Autodesk Fusion 360 part; units mm, degrees
(part 2 of 2)
sketch "bottom_shell" plane through (0, 0, -4.4) normal (0, 0, 1) x (1, 0, 0) in component "diag_up_bottom_noVM"
  circle A0 centre (49, 51) radius 1.5875 construction
  line L0 (1, 0) -> (52, 0) construction
  line L1 (0, 1) -> (0, 54) construction
  line L2 (53, 1) -> (53, 54) construction
  circle A1 centre (4, 51) radius 1.5875 construction
  line L3 (52, 55) -> (1, 55) construction
  line L4 (-7.5, 57.5) -> (60.5, 57.5)
  line L5 (63.5, 54.5) -> (63.5, 3)
  line L6 (60.5, 0) -> (-7.5, 0)
  line L7 (-10.5, 3) -> (-10.5, 54.5)
  arc A2 (-7.5, 57.5) -> (-10.5, 54.5) centre (-7.5, 54.5) ccw
  arc A3 (63.5, 54.5) -> (60.5, 57.5) centre (60.5, 54.5) ccw
  arc A4 (60.5, 0) -> (63.5, 3) centre (60.5, 3) ccw
  arc A5 (-10.5, 3) -> (-7.5, 0) centre (-7.5, 3) ccw
  arc A6 (61.5, 54.5) -> (60.5, 55.5) centre (60.5, 54.5) ccw
  line L8 (-7.5, 55.5) -> (60.5, 55.5)
  arc A7 (-7.5, 55.5) -> (-8.5, 54.5) centre (-7.5, 54.5) ccw
  line L9 (-8.5, 3) -> (-8.5, 54.5)
  arc A8 (-8.5, 3) -> (-7.5, 2) centre (-7.5, 3) ccw
  line L10 (60.5, 2) -> (-7.5, 2)
  arc A9 (60.5, 2) -> (61.5, 3) centre (60.5, 3) ccw
  line L11 (61.5, 54.5) -> (61.5, 3)
  arc A10 (62.3, 54.5) -> (60.5, 56.3) centre (60.5, 54.5) ccw
  line L12 (-7.5, 56.3) -> (60.5, 56.3)
  arc A11 (-7.5, 56.3) -> (-9.3, 54.5) centre (-7.5, 54.5) ccw
  line L13 (-9.3, 3) -> (-9.3, 54.5)
  arc A12 (-9.3, 3) -> (-7.5, 1.2) centre (-7.5, 3) ccw
  arc A13 (60.5, 1.2) -> (62.3, 3) centre (60.5, 3) ccw
  line L14 (62.3, 54.5) -> (62.3, 3)
  circle A14 centre (49, 51) radius 1.75
  circle A15 centre (49, 51) radius 3.5
  circle A16 centre (49, 51) radius 4.25
  circle A17 centre (4, 51) radius 1.75
  circle A18 centre (4, 51) radius 3.5
  circle A19 centre (4, 51) radius 4.25
  circle A20 centre (-4.25, 6.25) radius 1.75
  circle A21 centre (-4.25, 6.25) radius 3
  circle A22 centre (-4.25, 6.25) radius 4
  line L15 (-0.3, 2) -> (-0.3, 0)
  line L16 (53.3, 2) -> (53.3, 0)
  circle A23 centre (57.25, 6.25) radius 1.75
  circle A24 centre (57.25, 6.25) radius 3
  circle A25 centre (57.25, 6.25) radius 4
  line L17 (60.5, 1.2) -> (53, 1.2)
  line L18 (0, 1.2) -> (-7.5, 1.2)
  line L19 (26.5, 55) -> (26.5, 2) construction
  line L20 (-5.7027, 21) -> (58.2376, 21) construction
  line L21 (-2, 22.5) -> (2, 22.5)
  line L22 (2, 22.5) -> (2, 19.5)
  line L23 (2, 19.5) -> (-2, 19.5)
  line L24 (-2, 19.5) -> (-2, 22.5)
  line L25 (-0.3, 22.5) -> (-0.3, 19.5)
  line L26 (51, 22.5) -> (55, 22.5)
  line L27 (55, 22.5) -> (55, 19.5)
  line L28 (55, 19.5) -> (51, 19.5)
  line L29 (51, 19.5) -> (51, 22.5)
  line L30 (54, 22.5) -> (53.3, 22.5)
  line L31 (53.3, 22.5) -> (53.3, 19.5)
  line L32 (53.3, 19.5) -> (54, 19.5)
  line L33 (-8.5, 22.5) -> (-8.5, 22.5)
  line L34 (-2, 22.5) -> (-2, 22.5)
  line L35 (-2, 19.5) -> (-8.5, 19.5)
  line L36 (-8.5, 19.5) -> (-8.5, 19.5)
  line L37 (-2, 19.5) -> (-2, 19.5)
  line L38 (55, 22.5) -> (61.5, 22.5)
  line L39 (55, 19.5) -> (61.5, 19.5)
  line L40 (-2, 22.5) -> (-8.5, 22.5)
  line L41 (-4.25, 6.25) -> (-4.25, 10.25) construction
  line L42 (-4.25, 6.25) -> (-0.25, 6.25) construction
  line L43 (57.25, 6.25) -> (53.25, 6.25) construction
  line L44 (57.25, 6.25) -> (57.25, 10.25) construction
  line L45 (57.25, 10.25) -> (61.5, 10.25)
  line L46 (53.3, 2) -> (53.3, 5.6195)
  line L47 (-4.25, 10.25) -> (-8.5, 10.25)
  line L48 (4, 51) -> (8.25, 51) construction
  line L49 (4, 51) -> (-0.25, 51) construction
  line L50 (49, 51) -> (53.25, 51) construction
  line L51 (49, 51) -> (44.75, 51) construction
  line L52 (44.75, 51) -> (44.75, 55.5)
  line L53 (53.25, 51) -> (53.25, 55.5)
  line L54 (8.25, 51) -> (8.25, 55.5)
  line L55 (-0.25, 51) -> (-0.25, 55.5)
  line L56 (-0.3, 2) -> (-0.3, 5.6195)
  point P0 (49, 51)
  point P1 (49, 51)
  dimension "d47" = 57.5
  dimension "d48" = 3
  dimension "d49" = 10.5
  dimension "d50" = 74
  dimension "d51" = 2
  dimension "d53" = 3.5
  dimension "d54" = 7
  dimension "d56" = 3.5
  dimension "d57" = 7
  dimension "d58" = 8.5
  dimension "d59" = 4.25
  dimension "d60" = 4.25
  dimension "d61" = 3.5
  dimension "d62" = 6
  dimension "d63" = 8
  dimension "d64" = 0.3
  dimension "d65" = 0.3
  dimension "d66" = 3.5
  dimension "d67" = 4.25
  dimension "d68" = 4.25
  dimension "d69" = 6
  dimension "d70" = 8
  dimension "d71" = 8.5
  dimension "d72" = 1.2
  dimension "d85" = 19
  dimension "d86" = 4
  dimension "d87" = 3
  dimension "d88" = 0.3
  dimension "d89" = 4
  dimension "d90" = 3
  dimension "d91" = 0.3
  constraint horizontal L4
  constraint vertical L5
  constraint horizontal L6
  constraint vertical L7
  constraint collinear L0 L6
  constraint tangent L4 A2
  constraint tangent L7 A2
  constraint tangent L4 A3
  constraint tangent L5 A3
  constraint equal A2 A3
  constraint tangent L5 A4
  constraint tangent L6 A4
  constraint equal A2 A4
  constraint tangent L6 A5
  constraint tangent L7 A5
  constraint equal A2 A5
  constraint coincident P0 A0.centre
  constraint concentric A14 A15
  constraint concentric A15 A16
  constraint concentric A1 A17
  constraint concentric A1 A18
  constraint concentric A17 A19
  constraint concentric A20 A21
  constraint concentric A20 A22
  constraint coincident L10 L15.start
  constraint coincident L6 L15.end
  constraint perpendicular L6 L15
  constraint coincident L10 L16.start
  constraint coincident L6 L16.end
  constraint perpendicular L6 L16
  constraint concentric A23 A24
  constraint concentric A24 A25
  constraint concentric A3 A10
  constraint parallel L4 L12
  constraint concentric A2 A11
  constraint parallel L7 L13
  constraint concentric A5 A12
  constraint parallel L6 L17
  constraint concentric A4 A13
  constraint parallel L5 L14
  constraint tangent A10 L14
  constraint tangent A13 L17
  constraint tangent A10 L12
  constraint tangent A13 L14
  constraint tangent L12 A11
  constraint tangent A11 L13
  constraint tangent A12 L17
  constraint tangent L13 A12
  constraint coincident L2 L17.end
  constraint coincident L1 L18.start
  constraint collinear L17 L18
  constraint midpoint L3 L19.start
  constraint midpoint L10 L19.end
  constraint perpendicular L2 L20
  constraint horizontal L21
  constraint vertical L22
  constraint horizontal L23
  constraint vertical L24
  constraint symmetric L20 L21 L23
  constraint symmetric L1 L22 L24
  constraint coincident L21 L25.start
  constraint coincident L23 L25.end
  constraint perpendicular L23 L25
  constraint horizontal L26
  constraint vertical L27
  constraint horizontal L28
  constraint vertical L29
  constraint horizontal L30
  constraint vertical L31
  constraint horizontal L32
  constraint coincident L28 L31.end
  constraint coincident L26 L30.start
  constraint symmetric L20 L26 L28
  constraint symmetric L2 L27 L29
  constraint coincident L9 L33.start
  constraint horizontal L35
  constraint coincident L9 L35.end
  constraint coincident L11 L38.end
  constraint perpendicular L11 L38
  constraint coincident L11 L39.end
  constraint perpendicular L11 L39
  constraint perpendicular L9 L40
  constraint coincident A20.centre A21.centre
  constraint coincident A22 L41.end
  constraint vertical L41
  constraint coincident A22 L42.end
  constraint perpendicular L41 L42
  constraint coincident A23.centre A24.centre
  constraint coincident A25 L43.end
  constraint perpendicular L19 L43
  constraint coincident A25 L44.end
  constraint perpendicular L43 L44
  constraint coincident L11 L45.end
  constraint tangent A25 L45
  constraint coincident A25 L46.end
  constraint perpendicular L10 L46
  constraint coincident L9 L47.end
  constraint tangent A22 L47
  constraint coincident A1.centre A17.centre
  constraint coincident A19 L48.end
  constraint horizontal L48
  constraint coincident A19 L49.end
  constraint perpendicular L1 L49
  constraint coincident P1 P0
  constraint coincident A16 L50.end
  constraint coincident A16 L51.end
  constraint horizontal L51
  constraint coincident L8 L52.end
  constraint tangent A16 L52
  constraint coincident L8 L53.end
  constraint tangent A16 L53
  constraint perpendicular L8 L53
  constraint coincident L8 L54.end
  constraint tangent A19 L54
  constraint coincident L8 L55.end
  constraint tangent A19 L55
  constraint coincident A22 L56.end
  constraint perpendicular L10 L56
  measures "d47" distance of L4 L6
  measures "d48" radius of A2
  measures "d49" distance of L1 L7
  measures "d50" distance of L5 L7
  measures "d53" diameter of A14
  measures "d54" diameter of A15
  measures "d56" diameter of A17
  measures "d57" diameter of A18
  measures "d58" diameter of A19
  measures "d59" distance of L1 A20.centre
  measures "d60" distance of L10 A20.centre
  measures "d61" diameter of A20
  measures "d62" diameter of A21
  measures "d63" diameter of A22
  measures "d64" distance of L1 L15
  measures "d65" distance of L2 L16
  measures "d66" diameter of A23
  measures "d67" distance of L2 A23.centre
  measures "d68" distance of L10 A23.centre
  measures "d69" diameter of A24
  measures "d70" diameter of A25
  measures "d71" diameter of A16
  measures "d72" distance of L7 L13
  measures "d85" distance of L10 L20
  measures "d86" distance of L22 L24
  measures "d87" distance of L21 L23
  measures "d88" distance of L1 L25
  measures "d89" distance of L27 L29
  measures "d90" distance of L26 L28
  measures "d91" distance of L2 L31
extrude "Extrude1'" add sketch "bottom_shell" against normal blind 2 separate body contours L4 L5 L6 L7 A2 A3 A4 A5 A10 L12 A11 L13 A12 A13 L14 L15 L16 L17 L18 | L6 L10 L15 L16 | A6 L8 A7 L9 A8 L10 A9 L11 A10 L12 A11 L13 A12 A13 L14 L15 L16 L17 L18 | A6 L8 A7 L9 L10 L11 A16 A19 A22 A25 L21 L22 L23 L26 L28 L29 L30 L32 L35 L38 L39 L40 L45 L46 L47 L52 L53 L54 L55 L56 | L9 A8 L10 A22 L47 L56 | L10 A9 L11 A25 L45 L46 | A22 | A25 | L9 L24 L35 L40 | L11 L27 L38 L39 | L21 L23 L24 L25 | L26 L27 L28 L30 L31 L32 | L21 L22 L23 L25 | L26 L28 L29 L31 | L8 A19 L54 L55 | L8 A16 L52 L53 | A19 | A16 makes body 2 in component "diag_up_bottom_noVM"
extrude "Extrude2'" add sketch "bottom_shell" along normal blind 1 contours L6 L10 L15 L16 bodies 2 in component "diag_up_bottom_noVM"
extrude "Extrude3'" add sketch "bottom_shell" along normal blind 9.7 contours A6 L8 A7 L9 A8 L10 A9 L11 A10 L12 A11 L13 A12 A13 L14 L15 L16 L17 L18 bodies 2 in component "diag_up_bottom_noVM"
extrude "Extrude4'" add sketch "bottom_shell" along normal blind 8.7 contours L4 L5 L6 L7 A2 A3 A4 A5 A10 L12 A11 L13 A12 A13 L14 L15 L16 L17 L18 bodies 2 in component "diag_up_bottom_noVM"
extrude "Extrude5'" add sketch "bottom_shell" along normal blind 2.8 contours L21 L22 L23 L25 | L26 L28 L29 L31 | L8 A19 L54 L55 | L8 A16 L52 L53 | A19 | A16 | A15 | A18 bodies 2 in component "diag_up_bottom_noVM"
extrude "Extrude6'" add sketch "bottom_shell" along normal blind 4.4 contours L9 A8 L10 A22 L47 L56 | L10 A9 L11 A25 L45 L46 | A22 | A25 | L9 L24 L35 L40 | L11 L27 L38 L39 | L21 L23 L24 L25 | L26 L27 L28 L30 L31 L32 | A21 | A24 bodies 2 in component "diag_up_bottom_noVM"
fillet "Fillet6" radius 1 10 edges at (8.25, 55.5, -3) (-0.25, 55.5, -3) (-8.5, 22.5, -2.2) (-8.5, 19.5, -2.2) (-8.5, 10.25, -2.2) (61.5, 10.25, -2.2) (61.5, 19.5, -2.2) (61.5, 22.5, -2.2) (53.25, 55.5, -3) (44.75, 55.5, -3) on bodies 2 in component "diag_up_bottom_noVM"
chamfer "Chamfer2" distance 1 angle 45 18 edges at (-5.875, 10.25, 0) (-8.2071, 10.5429, 0) (-1.2068, 8.846, 0) (-0.3, 3.8098, 0) (4, 46.75, -1.6) (8.25, 52.75, -1.6) (8.5429, 55.2071, -1.6) (-0.5429, 55.2071, -1.6) (-0.25, 52.75, -1.6) (44.75, 52.75, -1.6) (49, 46.75, -1.6) (53.25, 52.75, -1.6) (53.5429, 55.2071, -1.6) (44.4571, 55.2071, -1.6) (58.875, 10.25, 0) (54.2068, 8.846, 0) (61.2071, 10.5429, 0) (53.3, 3.8098, 0) on bodies 2 in component "diag_up_bottom_noVM"
fillet "Fillet7" radius 0.5 8 edges at (-0.3, 22.5, -0.8) (2, 22.5, -3) (2, 19.5, -3) (-0.3, 19.5, -0.8) (53.3, 22.5, -0.8) (53.3, 19.5, -0.8) (51, 19.5, -3) (51, 22.5, -3) on bodies 2 in component "diag_up_bottom_noVM"
fillet "Fillet8" radius 0.5 42 edges at (54.2068, 8.846, -4.4) (58.875, 10.25, -4.4) (61.2071, 10.5429, -4.4) (61.5, 14.875, -4.4) (61.2071, 19.2071, -4.4) (56, 19.5, -4.4) (51.1464, 19.6464, -4.4) (51, 21, -4.4) (51.1464, 22.3536, -4.4) (56, 22.5, -4.4) (61.2071, 22.7929, -4.4) (61.5, 39, -4.4) (61.2071, 55.2071, -4.4) (57.375, 55.5, -4.4) (53.5429, 55.2071, -4.4) (53.25, 52.75, -4.4) (49, 46.75, -4.4) (44.75, 52.75, -4.4) (44.4571, 55.2071, -4.4) (26.5, 55.5, -4.4) (8.5429, 55.2071, -4.4) (8.25, 52.75, -4.4) (4, 46.75, -4.4) (-0.25, 52.75, -4.4) (-0.5429, 55.2071, -4.4) (-4.375, 55.5, -4.4) (-8.2071, 55.2071, -4.4) (-8.5, 39, -4.4) (-8.2071, 22.7929, -4.4) (-3, 22.5, -4.4) (1.8536, 22.3536, -4.4) (2, 21, -4.4) (1.8536, 19.6464, -4.4) (-3, 19.5, -4.4) (-8.2071, 19.2071, -4.4) (-8.5, 14.875, -4.4) (-8.2071, 10.5429, -4.4) (-5.875, 10.25, -4.4) (-1.2068, 8.846, -4.4) (-0.3, 3.8098, -4.4) (53.3, 3.8098, -4.4) (26.5, 2, -4.4) on bodies 2 in component "diag_up_bottom_noVM"
fillet "Fillet9" radius 0.5 3 edges at (-0.3, 0, 0.45) (26.5, 0, -3.4) (53.3, 0, 0.45) on bodies 2 in component "diag_up_bottom_noVM"
fillet "Fillet10" radius 0.5 2 edges at (-0.3, 2, 2.15) (53.3, 2, 2.15) on bodies 2 in component "diag_up_bottom_noVM"
fillet "Fillet11" radius 0.5 2 edges at (4, 55.5, -1.6) (49, 55.5, -1.6) on bodies 2 in component "diag_up_bottom_noVM"
fillet "Fillet12" radius 0.5 2 edges at (-8.5, 21, 0) (61.5, 21, 0) on bodies 2 in component "diag_up_bottom_noVM"
ref_plane "WorkPlane1" through (0, 0, 8) normal (0, 0, 1) x (1, 0, 0) in component "diag_up_top_noVM"
sketch "top shell" plane through (0, 0, 8) normal (0, 0, 1) x (1, 0, 0) in component "diag_up_top_noVM"
  line L0 (2.8575, 28.7338) -> (4.2862, 28.7338) construction
  line L1 (1.4287, 28.7338) -> (2.8575, 28.7338) construction
  line L2 (1.4287, 8.4138) -> (1.4287, 28.7338) construction
  line L3 (4.2862, 28.7338) -> (10.6363, 28.7338) construction
  line L4 (10.6363, 28.7338) -> (10.6363, 20.6376) construction
  line L5 (10.6363, 20.6376) -> (10.6363, 16.5099) construction
  line L6 (10.6363, 16.5099) -> (10.6363, 8.4138) construction
  line L7 (10.6363, 8.4138) -> (4.2862, 8.4138) construction
  line L8 (4.2862, 8.4138) -> (2.8575, 8.4138) construction
  line L9 (2.8575, 8.4138) -> (1.4287, 8.4138) construction
  line L10 (16.84, 48.2537) -> (16.84, 54.6038) construction
  line L11 (16.84, 54.6038) -> (24.9362, 54.6038) construction
  line L12 (16.84, 46.825) -> (16.84, 48.2537) construction
  line L13 (16.84, 45.3962) -> (16.84, 46.825) construction
  line L14 (37.16, 45.3962) -> (16.84, 45.3962) construction
  line L15 (37.16, 46.825) -> (37.16, 45.3962) construction
  line L16 (37.16, 48.2537) -> (37.16, 46.825) construction
  line L17 (37.16, 54.6038) -> (37.16, 48.2537) construction
  line L18 (29.0638, 54.6038) -> (37.16, 54.6038) construction
  line L19 (24.9362, 54.6038) -> (29.0638, 54.6038) construction
  line L20 (46.2537, 45.16) -> (52.6038, 45.16) construction
  line L21 (44.825, 45.16) -> (46.2537, 45.16) construction
  line L22 (43.3962, 45.16) -> (44.825, 45.16) construction
  line L23 (43.3962, 24.84) -> (43.3962, 45.16) construction
  line L24 (52.6038, 45.16) -> (52.6038, 37.0638) construction
  line L25 (52.6038, 37.0638) -> (52.6038, 32.9362) construction
  line L26 (52.6038, 32.9362) -> (52.6038, 24.84) construction
  line L27 (52.6038, 24.84) -> (46.2537, 24.84) construction
  line L28 (46.2537, 24.84) -> (44.825, 24.84) construction
  line L29 (44.825, 24.84) -> (43.3962, 24.84) construction
  line L30 (43.3962, 23.62) -> (44.825, 23.62) construction
  line L31 (44.825, 23.62) -> (46.2537, 23.62) construction
  line L32 (46.2537, 23.62) -> (52.6038, 23.62) construction
  line L33 (52.6038, 23.62) -> (52.6038, 17.27) construction
  line L34 (43.3962, 8.38) -> (43.3962, 23.62) construction
  line L35 (44.825, 8.38) -> (43.3962, 8.38) construction
  line L36 (46.2537, 8.38) -> (44.825, 8.38) construction
  line L37 (52.6038, 8.38) -> (46.2537, 8.38) construction
  line L38 (52.6038, 14.73) -> (52.6038, 8.38) construction
  line L39 (52.6038, 17.27) -> (52.6038, 14.73) construction
  circle A0 centre (49, 51) radius 1.5875 construction
  circle A1 centre (57.25, 6.25) radius 1.75 construction
  circle A2 centre (-4.25, 6.25) radius 1.75 construction
  circle A3 centre (4, 51) radius 1.5875 construction
  line L40 (0, 1) -> (0, 54) construction
  line L41 (53, 1) -> (53, 54) construction
  line L42 (60.5, 2) -> (-7.5, 2)
  line L43 (60.5, 0) -> (-7.5, 0)
  arc A4 (-10.5, 3) -> (-7.5, 0) centre (-7.5, 3) ccw
  arc A5 (-8.5, 3) -> (-7.5, 2) centre (-7.5, 3) ccw
  line L44 (-8.5, 3) -> (-8.5, 54.5)
  line L45 (-10.5, 3) -> (-10.5, 54.5)
  arc A6 (-7.5, 55.5) -> (-8.5, 54.5) centre (-7.5, 54.5) ccw
  arc A7 (-7.5, 57.5) -> (-10.5, 54.5) centre (-7.5, 54.5) ccw
  line L46 (-7.5, 57.5) -> (60.5, 57.5)
  line L47 (-7.5, 55.5) -> (60.5, 55.5)
  arc A8 (63.5, 54.5) -> (60.5, 57.5) centre (60.5, 54.5) ccw
  arc A9 (61.5, 54.5) -> (60.5, 55.5) centre (60.5, 54.5) ccw
  line L48 (63.5, 54.5) -> (63.5, 3)
  line L49 (61.5, 54.5) -> (61.5, 3)
  arc A10 (60.5, 0) -> (63.5, 3) centre (60.5, 3) ccw
  arc A11 (60.5, 2) -> (61.5, 3) centre (60.5, 3) ccw
  line L50 (0, 2) -> (0, 0)
  line L51 (53, 2) -> (53, 0)
  arc A12 (62.7, 54.5) -> (60.5, 56.7) centre (60.5, 54.5) ccw
  line L52 (-7.5, 56.7) -> (60.5, 56.7)
  arc A13 (-7.5, 56.7) -> (-9.7, 54.5) centre (-7.5, 54.5) ccw
  line L53 (-9.7, 3) -> (-9.7, 54.5)
  arc A14 (-9.7, 3) -> (-7.5, 0.8) centre (-7.5, 3) ccw
  arc A15 (60.5, 0.8) -> (62.7, 3) centre (60.5, 3) ccw
  line L54 (62.7, 54.5) -> (62.7, 3)
  line L55 (60.5, 0.8) -> (53, 0.8)
  line L56 (0, 0.8) -> (-7.5, 0.8)
  circle A16 centre (4, 51) radius 1.25
  circle A17 centre (57.25, 6.25) radius 1.25
  circle A18 centre (-4.25, 6.25) radius 1.25
  circle A19 centre (49, 51) radius 1.25
  circle A20 centre (4, 51) radius 3.5
  circle A21 centre (49, 51) radius 3.5
  circle A22 centre (57.25, 6.25) radius 3.5
  circle A23 centre (-4.25, 6.25) radius 3.5
  line L57 (16.74, 44.7962) -> (37.26, 44.7962)
  line L58 (37.76, 45.2962) -> (37.76, 54.7038)
  line L59 (37.26, 55.2038) -> (16.74, 55.2038)
  line L60 (16.24, 54.7038) -> (16.24, 45.2962)
  line L61 (10.7363, 7.8138) -> (1.3287, 7.8138)
  line L62 (0.8287, 8.3138) -> (0.8287, 28.8338)
  line L63 (1.3287, 29.3338) -> (10.7363, 29.3338)
  line L64 (11.2363, 28.8338) -> (11.2363, 8.3138)
  line L65 (43.2962, 7.78) -> (52.7038, 7.78)
  line L66 (53.2038, 8.28) -> (53.2038, 45.26)
  line L67 (52.7038, 45.76) -> (43.2962, 45.76)
  line L68 (42.7962, 45.26) -> (42.7962, 8.28)
  arc A24 (1.3287, 29.3338) -> (0.8287, 28.8338) centre (1.3287, 28.8338) ccw
  arc A25 (11.2363, 28.8338) -> (10.7363, 29.3338) centre (10.7363, 28.8338) ccw
  arc A26 (10.7363, 7.8138) -> (11.2363, 8.3138) centre (10.7363, 8.3138) ccw
  arc A27 (0.8287, 8.3138) -> (1.3287, 7.8138) centre (1.3287, 8.3138) ccw
  arc A28 (16.74, 55.2038) -> (16.24, 54.7038) centre (16.74, 54.7038) ccw
  arc A29 (16.24, 45.2962) -> (16.74, 44.7962) centre (16.74, 45.2962) ccw
  arc A30 (37.26, 44.7962) -> (37.76, 45.2962) centre (37.26, 45.2962) ccw
  arc A31 (37.76, 54.7038) -> (37.26, 55.2038) centre (37.26, 54.7038) ccw
  arc A32 (43.2962, 45.76) -> (42.7962, 45.26) centre (43.2962, 45.26) ccw
  arc A33 (53.2038, 45.26) -> (52.7038, 45.76) centre (52.7038, 45.26) ccw
  arc A34 (52.7038, 7.78) -> (53.2038, 8.28) centre (52.7038, 8.28) ccw
  arc A35 (42.7962, 8.28) -> (43.2962, 7.78) centre (43.2962, 8.28) ccw
  line L69 (32.6707, 18.161) -> (15.9068, 18.161) construction
  line L70 (32.6707, 18.161) -> (32.6707, 12.319) construction
  line L71 (15.9068, 12.319) -> (32.6707, 12.319) construction
  line L72 (15.9068, 12.319) -> (15.9068, 14.224) construction
  line L73 (15.9068, 18.161) -> (15.9068, 16.256) construction
  line L74 (15.9068, 22.6378) -> (32.6707, 22.6378) construction
  line L75 (32.6707, 28.4798) -> (32.6707, 22.6378) construction
  line L76 (32.6707, 28.4798) -> (15.9068, 28.4798) construction
  line L77 (15.9068, 28.4798) -> (15.9068, 26.5748) construction
  line L78 (15.9068, 22.6378) -> (15.9068, 24.5428) construction
  line L79 (15.9068, 32.9565) -> (32.6707, 32.9565) construction
  line L80 (32.6707, 38.7985) -> (32.6707, 32.9565) construction
  line L81 (32.6707, 38.7985) -> (15.9068, 38.7985) construction
  line L82 (15.9068, 38.7985) -> (15.9068, 36.8935) construction
  line L83 (15.9068, 32.9565) -> (15.9068, 34.8615) construction
  line L84 (15.9068, 39.7985) -> (32.6707, 39.7985)
  line L85 (33.6707, 38.7985) -> (33.6707, 32.9565)
  line L86 (32.6707, 31.9565) -> (15.9068, 31.9565)
  line L87 (14.9068, 32.9565) -> (14.9068, 38.7985)
  line L88 (15.9068, 29.4798) -> (32.6707, 29.4798)
  line L89 (33.6707, 28.4798) -> (33.6707, 22.6378)
  line L90 (32.6707, 21.6378) -> (15.9068, 21.6378)
  line L91 (14.9068, 22.6378) -> (14.9068, 28.4798)
  line L92 (15.9068, 19.161) -> (32.6707, 19.161)
  line L93 (33.6707, 18.161) -> (33.6707, 12.319)
  line L94 (32.6707, 11.319) -> (15.9068, 11.319)
  line L95 (14.9068, 12.319) -> (14.9068, 18.161)
  arc A36 (14.9068, 12.319) -> (15.9068, 11.319) centre (15.9068, 12.319) ccw
  arc A37 (32.6707, 11.319) -> (33.6707, 12.319) centre (32.6707, 12.319) ccw
  arc A38 (33.6707, 18.161) -> (32.6707, 19.161) centre (32.6707, 18.161) ccw
  arc A39 (15.9068, 19.161) -> (14.9068, 18.161) centre (15.9068, 18.161) ccw
  arc A40 (33.6707, 28.4798) -> (32.6707, 29.4798) centre (32.6707, 28.4798) ccw
  arc A41 (15.9068, 29.4798) -> (14.9068, 28.4798) centre (15.9068, 28.4798) ccw
  arc A42 (14.9068, 22.6378) -> (15.9068, 21.6378) centre (15.9068, 22.6378) ccw
  arc A43 (32.6707, 21.6378) -> (33.6707, 22.6378) centre (32.6707, 22.6378) ccw
  arc A44 (33.6707, 38.7985) -> (32.6707, 39.7985) centre (32.6707, 38.7985) ccw
  arc A45 (32.6707, 31.9565) -> (33.6707, 32.9565) centre (32.6707, 32.9565) ccw
  arc A46 (14.9068, 32.9565) -> (15.9068, 31.9565) centre (15.9068, 32.9565) ccw
  arc A47 (15.9068, 39.7985) -> (14.9068, 38.7985) centre (15.9068, 38.7985) ccw
  line L96 (0.5, 51) -> (0.5, 55.5)
  line L97 (7.5, 55.5) -> (7.5, 51)
  line L98 (45.5, 55.5) -> (45.5, 51)
  line L99 (52.5, 55.5) -> (52.5, 51)
  line L100 (53.75, 2) -> (53.75, 6.25)
  line L101 (61.5, 9.75) -> (57.25, 9.75)
  line L102 (-0.75, 2) -> (-0.75, 6.25)
  line L103 (-8.5, 9.75) -> (-4.25, 9.75)
  line L104 (4.445, 35.7188) -> (2.54, 35.7188) construction
  line L105 (2.54, 35.7188) -> (2.54, 33.8137) construction
  line L106 (3.175, 30.6388) -> (4.445, 30.6388) construction
  line L107 (5.08, 31.2738) -> (5.08, 32.5438) construction
  line L108 (8.0962, 52.705) -> (8.0962, 51.435) construction
  line L109 (8.7313, 50.8) -> (10.0013, 50.8) construction
  line L110 (15.7163, 53.34) -> (13.8113, 53.34) construction
  line L111 (15.7163, 51.435) -> (15.7163, 53.34) construction
  circle A48 centre (7.5, 45) radius 1.5 construction
  circle A49 centre (13, 45) radius 1.5 construction
  circle A50 centre (7.5, 45) radius 1.75
  circle A51 centre (13, 45) radius 1.75
  line L112 (8.0962, 50.5) -> (16.24, 50.5)
  line L113 (16.24, 50.5) -> (16.24, 53.64)
  line L114 (16.24, 53.64) -> (8.0962, 53.64)
  line L115 (7.7962, 53.34) -> (7.7962, 50.8)
  line L116 (2.54, 36.0188) -> (5.08, 36.0188)
  line L117 (5.38, 35.7188) -> (5.38, 30.6388)
  line L118 (5.08, 30.3388) -> (2.54, 30.3388)
  line L119 (2.24, 30.6388) -> (2.24, 35.7188)
  arc A52 (5.38, 35.7188) -> (5.08, 36.0188) centre (5.08, 35.7188) ccw
  arc A53 (2.54, 36.0188) -> (2.24, 35.7188) centre (2.54, 35.7188) ccw
  arc A54 (2.24, 30.6388) -> (2.54, 30.3388) centre (2.54, 30.6388) ccw
  arc A55 (5.08, 30.3388) -> (5.38, 30.6388) centre (5.08, 30.6388) ccw
  arc A56 (8.0962, 53.64) -> (7.7962, 53.34) centre (8.0962, 53.34) ccw
  arc A57 (7.7962, 50.8) -> (8.0962, 50.5) centre (8.0962, 50.8) ccw
  dimension "d100" = 0.8
  dimension "d101" = 2.5
  dimension "d102" = 2.5
  dimension "d103" = 2.5
  dimension "d104" = 2.5
  dimension "d105" = 7
  dimension "d106" = 7
  dimension "d107" = 7
  dimension "d108" = 7
  dimension "d109" = 0.6
  dimension "d110" = 0.6
  dimension "d111" = 0.6
  dimension "d112" = 0.6
  dimension "d113" = 0.6
  dimension "d114" = 0.6
  dimension "d115" = 0.6
  dimension "d116" = 0.6
  dimension "d117" = 0.6
  dimension "d118" = 0.6
  dimension "d119" = 0.6
  dimension "d120" = 0.6
  dimension "d121" = 0.5
  dimension "d122" = 0.5
  dimension "d123" = 0.5
  dimension "d142" = 1
  dimension "d143" = 1
  dimension "d144" = 1
  dimension "d145" = 1
  dimension "d146" = 1
  dimension "d147" = 1
  dimension "d148" = 1
  dimension "d149" = 1
  dimension "d152" = 1
  dimension "d192" = 3.5
  dimension "d193" = 3.5
  dimension "d194" = 0.3
  dimension "d195" = 0.3
  dimension "d196" = 0.3
  dimension "d198" = 0.3
  dimension "d199" = 0.3
  dimension "d200" = 0.3
  dimension "d201" = 0.3
  dimension "d202" = 0.3
  dimension "d203" = 0.3
  constraint coincident L42 L50.start
  constraint coincident L40 L50.start
  constraint coincident L50.end origin
  constraint coincident L42 L51.start
  constraint coincident L41 L51.start
  constraint coincident L43 L51.end
  constraint perpendicular L43 L51
  constraint concentric A8 A12
  constraint parallel L46 L52
  constraint concentric A7 A13
  constraint parallel L45 L53
  constraint concentric A4 A14
  constraint parallel L43 L55
  constraint concentric A10 A15
  constraint parallel L48 L54
  constraint tangent A15 L54
  constraint tangent L53 A14
  constraint tangent A12 L54
  constraint tangent A12 L52
  constraint tangent L52 A13
  constraint tangent A13 L53
  constraint tangent A15 L55
  constraint tangent A14 L55
  constraint coincident L51 L55.end
  constraint coincident L50 L56.start
  constraint collinear L55 L56
  constraint concentric A3 A16
  constraint concentric A1 A17
  constraint concentric A2 A18
  constraint concentric A0 A19
  constraint concentric A16 A20
  constraint concentric A19 A21
  constraint concentric A17 A22
  constraint concentric A18 A23
  constraint horizontal L57
  constraint vertical L58
  constraint horizontal L59
  constraint vertical L60
  constraint horizontal L61
  constraint vertical L62
  constraint horizontal L63
  constraint vertical L64
  constraint horizontal L65
  constraint vertical L66
  constraint horizontal L67
  constraint vertical L68
  constraint tangent L62 A24
  constraint tangent L63 A24
  constraint tangent L63 A25
  constraint tangent L64 A25
  constraint equal A24 A25
  constraint tangent L61 A26
  constraint tangent L64 A26
  constraint equal A24 A26
  constraint tangent L61 A27
  constraint tangent L62 A27
  constraint equal A24 A27
  constraint tangent L59 A28
  constraint tangent L60 A28
  constraint tangent L57 A29
  constraint tangent L60 A29
  constraint equal A28 A29
  constraint tangent L57 A30
  constraint tangent L58 A30
  constraint equal A28 A30
  constraint tangent L58 A31
  constraint tangent L59 A31
  constraint equal A28 A31
  constraint tangent L67 A32
  constraint tangent L68 A32
  constraint tangent L66 A33
  constraint tangent L67 A33
  constraint equal A32 A33
  constraint tangent L65 A34
  constraint tangent L66 A34
  constraint equal A32 A34
  constraint tangent L65 A35
  constraint tangent L68 A35
  constraint equal A32 A35
  constraint horizontal L84
  constraint vertical L85
  constraint horizontal L86
  constraint vertical L87
  constraint horizontal L88
  constraint vertical L89
  constraint horizontal L90
  constraint vertical L91
  constraint horizontal L92
  constraint vertical L93
  constraint horizontal L94
  constraint vertical L95
  constraint collinear L87 L91
  constraint collinear L91 L95
  constraint collinear L85 L89
  constraint collinear L89 L93
  constraint tangent L94 A36
  constraint tangent L95 A36
  constraint tangent L93 A37
  constraint tangent L94 A37
  constraint equal A36 A37
  constraint tangent L92 A38
  constraint tangent L93 A38
  constraint equal A36 A38
  constraint tangent L92 A39
  constraint tangent L95 A39
  constraint equal A36 A39
  constraint tangent L88 A40
  constraint tangent L89 A40
  constraint equal A36 A40
  constraint tangent L88 A41
  constraint tangent L91 A41
  constraint equal A36 A41
  constraint tangent L90 A42
  constraint tangent L91 A42
  constraint equal A36 A42
  constraint tangent L89 A43
  constraint tangent L90 A43
  constraint equal A36 A43
  constraint tangent L84 A44
  constraint tangent L85 A44
  constraint equal A36 A44
  constraint tangent L85 A45
  constraint tangent L86 A45
  constraint equal A36 A45
  constraint tangent L86 A46
  constraint tangent L87 A46
  constraint equal A36 A46
  constraint tangent L84 A47
  constraint tangent L87 A47
  constraint equal A36 A47
  constraint coincident L47 L96.end
  constraint perpendicular L47 L96
  constraint tangent A20 L96
  constraint coincident A20 L96.start
  constraint coincident L47 L97.start
  constraint perpendicular L47 L97
  constraint tangent A20 L97
  constraint coincident A20 L97.end
  constraint coincident L47 L98.start
  constraint perpendicular L47 L98
  constraint coincident L47 L99.start
  constraint perpendicular L47 L99
  constraint tangent A21 L98
  constraint tangent A21 L99
  constraint coincident A21 L98.end
  constraint coincident A21 L99.end
  constraint coincident L42 L100.start
  constraint perpendicular L42 L100
  constraint coincident L49 L101.start
  constraint perpendicular L49 L101
  constraint tangent A22 L100
  constraint tangent A22 L101
  constraint coincident L42 L102.start
  constraint perpendicular L42 L102
  constraint coincident L44 L103.start
  constraint perpendicular L44 L103
  constraint tangent A23 L103
  constraint tangent A23 L102
  constraint coincident A23 L103.end
  constraint coincident A23 L102.end
  constraint coincident A22 L100.end
  constraint coincident A22 L101.end
  constraint concentric A48 A50
  constraint concentric A49 A51
  constraint horizontal L112
  constraint vertical L113
  constraint horizontal L114
  constraint vertical L115
  constraint horizontal L116
  constraint vertical L117
  constraint horizontal L118
  constraint vertical L119
  constraint tangent L116 A52
  constraint tangent L117 A52
  constraint tangent L116 A53
  constraint tangent L119 A53
  constraint equal A52 A53
  constraint tangent L118 A54
  constraint tangent L119 A54
  constraint equal A52 A54
  constraint tangent L117 A55
  constraint tangent L118 A55
  constraint equal A52 A55
  constraint collinear L60 L113
  constraint tangent L114 A56
  constraint tangent L115 A56
  constraint tangent L112 A57
  constraint tangent L115 A57
  constraint equal A56 A57
  measures "d100" distance of L46 L52
  measures "d101" diameter of A16
  measures "d102" diameter of A17
  measures "d103" diameter of A18
  measures "d104" diameter of A19
  measures "d105" diameter of A20
  measures "d106" diameter of A21
  measures "d107" diameter of A22
  measures "d108" diameter of A23
  measures "d109" distance of L11 L59
  measures "d110" distance of L14 L57
  measures "d111" distance of L13 L60
  measures "d112" distance of L15 L58
  measures "d113" distance of L22 L67
  measures "d114" distance of L23 L68
  measures "d115" distance of L24 L66
  measures "d116" distance of L37 L65
  measures "d117" distance of L3 L63
  measures "d118" distance of L4 L64
  measures "d119" distance of L2 L62
  measures "d120" distance of L7 L61
  measures "d121" radius of A24
  measures "d122" radius of A28
  measures "d123" radius of A32
  measures "d142" distance of L82 L87
  measures "d143" distance of L80 L85
  measures "d144" distance of L81 L84
  measures "d145" distance of L79 L86
  measures "d146" distance of L76 L88
  measures "d147" distance of L74 L90
  measures "d148" distance of L69 L92
  measures "d149" distance of L71 L94
  measures "d152" radius of A36
  measures "d192" diameter of A50
  measures "d193" diameter of A51
  measures "d194" distance of L109 L112
  measures "d195" distance of L110 L114
  measures "d196" distance of L108 L115
  measures "d198" distance of L106 L118
  measures "d199" distance of L104 L116
  measures "d200" distance of L105 L119
  measures "d201" distance of L107 L117
  measures "d202" radius of A52
  measures "d203" radius of A56
extrude "Extrude1''" add sketch "top shell" along normal blind 1.3 separate body contours L42 A5 L44 A6 L47 A9 L49 A11 L50 L51 A12 L52 A13 L53 A14 A15 L54 L55 L56 | L42 L49 A11 A22 L100 L101 | L42 L44 A6 L47 A9 L49 A20 A21 A22 A23 L96 L97 L98 L99 L100 L101 L102 L103 | L42 L43 L50 L51 | A22 | L43 A4 L45 A7 L46 A8 L48 A10 L50 L51 A12 L52 A13 L53 A14 A15 L54 L55 L56 | L42 A5 L44 A23 L102 L103 | A23 | L47 A21 L98 L99 | A21 | L47 A20 L96 L97 | A20 | A16 | A17 | A18 | A19 | L84 L85 L86 L87 A44 A45 A46 A47 | L88 L89 L90 L91 A40 A41 A42 A43 | L92 L93 L94 L95 A36 A37 A38 A39 makes body 3 in component "diag_up_top_noVM"
extrude "Extrude7'" cut sketch "top shell" along normal blind 1 contours L84 L85 L86 L87 A44 A45 A46 A47 | L88 L89 L90 L91 A40 A41 A42 A43 | L92 L93 L94 L95 A36 A37 A38 A39 bodies 3 in component "diag_up_top_noVM"
extrude "Extrude2''" add sketch "top shell" against normal blind 7.8 contours A21 | A20 bodies 3 in component "diag_up_top_noVM"
extrude "Extrude3''" add sketch "top shell" against normal blind 7.8 contours A22 | A23 bodies 3 in component "diag_up_top_noVM"
extrude "Extrude4''" add sketch "top shell" against normal blind 2.5 contours L42 A5 L44 A6 L47 A9 L49 A11 L50 L51 A12 L52 A13 L53 A14 A15 L54 L55 L56 | L42 L49 A11 A22 L100 L101 | L42 A5 L44 A23 L102 L103 | L47 A21 L98 L99 | L47 A20 L96 L97 bodies 3 in component "diag_up_top_noVM"
extrude "Extrude5''" add sketch "top shell" against normal blind 3.5 contours L43 A4 L45 A7 L46 A8 L48 A10 L50 L51 A12 L52 A13 L53 A14 A15 L54 L55 L56 bodies 3 in component "diag_up_top_noVM"
extrude "Extrude6''" add sketch "top shell" against normal blind 5 contours L42 L43 L50 L51 bodies 3 in component "diag_up_top_noVM"
fillet "Fillet7'" radius 0.8 8 edges at (-8.5, 9.75, 6.75) (-0.75, 2, 6.75) (7.5, 55.5, 6.75) (0.5, 55.5, 6.75) (45.5, 55.5, 6.75) (52.5, 55.5, 6.75) (61.5, 9.75, 6.75) (53.75, 2, 6.75) on bodies 3 in component "diag_up_top_noVM"
fillet "Fillet8'" radius 0.5 4 edges at (4, 54.5, 5.5) (-6.7249, 3.7751, 5.5) (49, 54.5, 5.5) (59.7249, 3.7751, 5.5) on bodies 3 in component "diag_up_top_noVM"
fillet "Fillet1'" radius 2 8 edges at (63.5, 28.75, 9.3) (62.6213, 56.6213, 9.3) (26.5, 57.5, 9.3) (-9.6213, 56.6213, 9.3) (-10.5, 28.75, 9.3) (-9.6213, 0.8787, 9.3) (26.5, 0, 9.3) (62.6213, 0.8787, 9.3) on bodies 3 in component "diag_up_top_noVM"
fillet "Fillet9'" radius 0.5 28 edges at (-0.75, 4.525, 8) (-1.7751, 8.7249, 8) (-5.975, 9.75, 8) (-8.2657, 9.9843, 8) (-8.5, 32.525, 8) (-8.2071, 55.2071, 8) (-3.9, 55.5, 8) (0.2657, 55.2657, 8) (0.5, 52.85, 8) (4, 47.5, 8) (7.5, 52.85, 8) (7.7343, 55.2657, 8) (26.5, 55.5, 8) (45.2657, 55.2657, 8) (45.5, 52.85, 8) (49, 47.5, 8) (52.5, 52.85, 8) (52.7343, 55.2657, 8) (56.9, 55.5, 8) (61.2071, 55.2071, 8) (61.5, 32.525, 8) (61.2657, 9.9843, 8) (58.975, 9.75, 8) (54.7751, 8.7249, 8) (53.75, 4.525, 8) (53.5157, 2.2343, 8) (26.5, 2, 8) (-0.5157, 2.2343, 8) on bodies 3 in component "diag_up_top_noVM"
fillet "Fillet6'" radius 0.5 24 edges at (33.6707, 15.24, 9) (33.3778, 18.8681, 9) (24.2887, 19.161, 9) (15.1997, 18.8681, 9) (14.9068, 15.24, 9) (15.1997, 11.6119, 9) (24.2888, 11.319, 9) (33.3778, 11.6119, 9) (33.6707, 25.5588, 9) (33.3778, 29.1869, 9) (24.2887, 29.4798, 9) (15.1997, 29.1869, 9) (14.9068, 25.5588, 9) (15.1997, 21.9307, 9) (24.2887, 21.6378, 9) (33.3778, 21.9307, 9) (33.6707, 35.8775, 9) (33.3778, 39.5056, 9) (24.2887, 39.7985, 9) (15.1997, 39.5056, 9) (14.9068, 35.8775, 9) (15.1997, 32.2494, 9) (24.2888, 31.9565, 9) (33.3778, 32.2494, 9) on bodies 3 in component "diag_up_top_noVM"
fillet "Fillet10'" radius 0.5 2 edges at (16.24, 53.64, 8.65) (16.24, 50.5, 8.65) on bodies 3 in component "diag_up_top_noVM"
sketch "label outline" plane through (0, 0, 9.3) normal (0, 0, 1) x (-1, 0, 0) in component "Label"
  arc A0 (-16.24, -50) -> (-15.74, -50.5) centre (-15.74, -50) ccw construction
  line L0 (-15.74, -50.5) -> (-8.0962, -50.5) construction
  arc A1 (-7.7962, -50.8) -> (-8.0962, -50.5) centre (-8.0962, -50.8) ccw construction
  line L1 (-7.7962, -50.8) -> (-7.7962, -53.34) construction
  arc A2 (-8.0962, -53.64) -> (-7.7962, -53.34) centre (-8.0962, -53.34) ccw construction
  line L2 (-8.0962, -53.64) -> (-15.74, -53.64) construction
  arc A3 (-15.74, -53.64) -> (-16.24, -54.14) centre (-15.74, -54.14) ccw construction
  line L3 (-16.24, -54.14) -> (-16.24, -54.7038) construction
  arc A4 (-16.74, -55.2038) -> (-16.24, -54.7038) centre (-16.74, -54.7038) ccw construction
  line L4 (-16.74, -55.2038) -> (-37.26, -55.2038) construction
  arc A5 (-37.76, -54.7038) -> (-37.26, -55.2038) centre (-37.26, -54.7038) ccw construction
  line L5 (-37.76, -54.7038) -> (-37.76, -45.2962) construction
  arc A6 (-37.26, -44.7962) -> (-37.76, -45.2962) centre (-37.26, -45.2962) ccw construction
  line L6 (-37.26, -44.7962) -> (-16.74, -44.7962) construction
  arc A7 (-16.24, -45.2962) -> (-16.74, -44.7962) centre (-16.74, -45.2962) ccw construction
  line L7 (-16.24, -45.2962) -> (-16.24, -50) construction
  line L8 (-61.5, -3) -> (-61.5, -54.5) construction
  arc A8 (-61.5, -54.5) -> (-60.5, -55.5) centre (-60.5, -54.5) ccw construction
  line L9 (-60.5, -55.5) -> (7.5, -55.5) construction
  arc A9 (7.5, -55.5) -> (8.5, -54.5) centre (7.5, -54.5) ccw construction
  line L10 (8.5, -54.5) -> (8.5, -3) construction
  arc A10 (8.5, -3) -> (7.5, -2) centre (7.5, -3) ccw construction
  line L11 (7.5, -2) -> (-60.5, -2) construction
  arc A11 (-60.5, -2) -> (-61.5, -3) centre (-60.5, -3) ccw construction
  circle A12 centre (-7.5, -45) radius 1.75 construction
  circle A13 centre (-13, -45) radius 1.75 construction
  arc A14 (-42.7962, -8.28) -> (-43.2962, -7.78) centre (-43.2962, -8.28) ccw construction
  line L12 (-42.7962, -8.28) -> (-42.7962, -45.26) construction
  arc A15 (-43.2962, -45.76) -> (-42.7962, -45.26) centre (-43.2962, -45.26) ccw construction
  line L13 (-43.2962, -45.76) -> (-52.7038, -45.76) construction
  arc A16 (-53.2038, -45.26) -> (-52.7038, -45.76) centre (-52.7038, -45.26) ccw construction
  line L14 (-53.2038, -45.26) -> (-53.2038, -8.28) construction
  arc A17 (-52.7038, -7.78) -> (-53.2038, -8.28) centre (-52.7038, -8.28) ccw construction
  line L15 (-52.7038, -7.78) -> (-43.2962, -7.78) construction
  arc A18 (-2.24, -30.6388) -> (-2.54, -30.3388) centre (-2.54, -30.6388) ccw construction
  line L16 (-2.24, -30.6388) -> (-2.24, -35.7188) construction
  arc A19 (-2.54, -36.0188) -> (-2.24, -35.7188) centre (-2.54, -35.7188) ccw construction
  line L17 (-2.54, -36.0188) -> (-5.08, -36.0188) construction
  arc A20 (-5.38, -35.7188) -> (-5.08, -36.0188) centre (-5.08, -35.7188) ccw construction
  line L18 (-5.38, -35.7188) -> (-5.38, -30.6388) construction
  arc A21 (-5.08, -30.3388) -> (-5.38, -30.6388) centre (-5.08, -30.6388) ccw construction
  line L19 (-5.08, -30.3388) -> (-2.54, -30.3388) construction
  arc A22 (-1.3287, -29.3338) -> (-0.8287, -28.8338) centre (-1.3287, -28.8338) ccw construction
  line L20 (-1.3287, -29.3338) -> (-10.7363, -29.3338) construction
  arc A23 (-11.2363, -28.8338) -> (-10.7363, -29.3338) centre (-10.7363, -28.8338) ccw construction
  line L21 (-11.2363, -28.8338) -> (-11.2363, -8.3138) construction
  arc A24 (-10.7363, -7.8138) -> (-11.2363, -8.3138) centre (-10.7363, -8.3138) ccw construction
  line L22 (-10.7363, -7.8138) -> (-1.3287, -7.8138) construction
  arc A25 (-0.8287, -8.3138) -> (-1.3287, -7.8138) centre (-1.3287, -8.3138) ccw construction
  line L23 (-0.8287, -8.3138) -> (-0.8287, -28.8338) construction
  line L24 (7.5, -2.3) -> (-60.5, -2.3)
  arc A26 (-60.5, -2.3) -> (-61.2, -3) centre (-60.5, -3) ccw
  line L25 (-61.2, -3) -> (-61.2, -54.5)
  arc A27 (-61.2, -54.5) -> (-60.5, -55.2) centre (-60.5, -54.5) ccw
  arc A28 (7.5, -55.2) -> (8.2, -54.5) centre (7.5, -54.5) ccw
  line L26 (8.2, -54.5) -> (8.2, -3)
  arc A29 (8.2, -3) -> (7.5, -2.3) centre (7.5, -3) ccw
  arc A30 (-11.5363, -28.8338) -> (-10.7363, -29.6338) centre (-10.7363, -28.8338) ccw
  arc A31 (-1.3287, -29.6338) -> (-0.5287, -28.8338) centre (-1.3287, -28.8338) ccw
  line L27 (-0.5287, -8.3138) -> (-0.5287, -28.8338)
  arc A32 (-0.5287, -8.3138) -> (-1.3287, -7.5138) centre (-1.3287, -8.3138) ccw
  line L28 (-10.7363, -7.5138) -> (-1.3287, -7.5138)
  arc A33 (-10.7363, -7.5138) -> (-11.5363, -8.3138) centre (-10.7363, -8.3138) ccw
  line L29 (-11.5363, -28.8338) -> (-11.5363, -8.3138)
  arc A34 (-5.68, -35.7188) -> (-5.08, -36.3188) centre (-5.08, -35.7188) ccw
  line L30 (-2.54, -36.3188) -> (-5.08, -36.3188)
  arc A35 (-2.54, -36.3188) -> (-1.94, -35.7188) centre (-2.54, -35.7188) ccw
  line L31 (-1.94, -30.6388) -> (-1.94, -35.7188)
  line L32 (-5.68, -35.7188) -> (-5.68, -30.6388)
  circle A36 centre (-7.5, -45) radius 2.05
  circle A37 centre (-13, -45) radius 2.05
  line L33 (-38.06, -54.7038) -> (-38.06, -45.2962)
  arc A38 (-37.26, -44.4962) -> (-38.06, -45.2962) centre (-37.26, -45.2962) ccw
  line L34 (-37.26, -44.4962) -> (-16.74, -44.4962)
  arc A39 (-15.94, -45.2962) -> (-16.74, -44.4962) centre (-16.74, -45.2962) ccw
  line L35 (-15.94, -45.2962) -> (-15.94, -50)
  arc A40 (-15.94, -50) -> (-15.74, -50.2) centre (-15.74, -50) ccw
  line L36 (-15.74, -50.2) -> (-8.0962, -50.2)
  arc A41 (-7.4962, -50.8) -> (-8.0962, -50.2) centre (-8.0962, -50.8) ccw
  arc A42 (-15.74, -53.94) -> (-15.94, -54.14) centre (-15.74, -54.14) ccw construction
  arc A43 (-53.5038, -45.26) -> (-52.7038, -46.06) centre (-52.7038, -45.26) ccw
  line L37 (-43.2962, -46.06) -> (-52.7038, -46.06)
  arc A44 (-43.2962, -46.06) -> (-42.4962, -45.26) centre (-43.2962, -45.26) ccw
  line L38 (-42.4962, -8.28) -> (-42.4962, -45.26)
  arc A45 (-42.4962, -8.28) -> (-43.2962, -7.48) centre (-43.2962, -8.28) ccw
  line L39 (-52.7038, -7.48) -> (-43.2962, -7.48)
  arc A46 (-52.7038, -7.48) -> (-53.5038, -8.28) centre (-52.7038, -8.28) ccw
  line L40 (-53.5038, -45.26) -> (-53.5038, -8.28)
  line L41 (-1.94, -30.6388) -> (-1.94, -29.9338)
  line L42 (-5.68, -30.6388) -> (-5.68, -29.9338)
  line L43 (-1.3287, -29.6338) -> (-1.64, -29.6338)
  line L44 (-5.98, -29.6338) -> (-10.7363, -29.6338)
  arc A47 (-1.64, -29.6338) -> (-1.94, -29.9338) centre (-1.64, -29.9338) ccw
  arc A48 (-5.68, -29.9338) -> (-5.98, -29.6338) centre (-5.98, -29.9338) ccw
  line L45 (-38.06, -54.7038) -> (-38.06, -54.7)
  line L46 (-7.4962, -50.8) -> (-7.4962, -54.7)
  line L47 (-60.5, -55.2) -> (-38.56, -55.2)
  line L48 (-6.9962, -55.2) -> (7.5, -55.2)
  arc A49 (-7.4962, -54.7) -> (-6.9962, -55.2) centre (-6.9962, -54.7) ccw
  arc A50 (-38.56, -55.2) -> (-38.06, -54.7) centre (-38.56, -54.7) ccw
  dimension "d209" = 0.3
  dimension "d210" = 0.3
  dimension "d212" = -0.3
  dimension "d213" = 0.3
  dimension "d214" = 0.3
  dimension "d215" = 0.3
  dimension "d216" = 0.3
  dimension "d217" = 0.3
  dimension "d218" = 0.5
  constraint concentric A20 A34
  constraint parallel L17 L30
  constraint concentric A19 A35
  constraint parallel L16 L31
  constraint parallel L18 L32
  constraint tangent A34 L32
  constraint tangent A34 L30
  constraint tangent L30 A35
  constraint tangent A35 L31
  constraint perpendicular L41 L43
  constraint perpendicular L42 L43
  constraint concentric A23 A30
  constraint parallel L20 L43
  constraint concentric A22 A31
  constraint parallel L23 L27
  constraint concentric A25 A32
  constraint parallel L22 L28
  constraint concentric A24 A33
  constraint parallel L21 L29
  constraint tangent L28 A33
  constraint tangent A30 L29
  constraint tangent A30 L43
  constraint tangent A33 L29
  constraint tangent A31 L43
  constraint tangent A31 L27
  constraint tangent A32 L28
  constraint tangent L27 A32
  constraint collinear L43 L44
  constraint tangent L41 A47
  constraint tangent L43 A47
  constraint tangent L42 A48
  constraint tangent L44 A48
  constraint equal A47 A48
  constraint parallel L5 L33
  constraint concentric A6 A38
  constraint parallel L6 L34
  constraint concentric A7 A39
  constraint parallel L7 L35
  constraint concentric A0 A40
  constraint parallel L0 L36
  constraint concentric A1 A41
  constraint concentric A3 A42
  constraint tangent L34 A39
  constraint tangent L33 A38
  constraint tangent A38 L34
  constraint tangent A39 L35
  constraint tangent L35 A40
  constraint tangent A40 L36
  constraint tangent L36 A41
  constraint perpendicular L45 L47
  constraint tangent A41 L46
  constraint perpendicular L46 L47
  constraint parallel L11 L24
  constraint concentric A11 A26
  constraint parallel L8 L25
  constraint concentric A8 A27
  constraint parallel L9 L47
  constraint concentric A9 A28
  constraint parallel L10 L26
  constraint concentric A10 A29
  constraint tangent A28 L26
  constraint tangent L24 A29
  constraint tangent L24 A26
  constraint tangent A26 L25
  constraint tangent A27 L47
  constraint tangent L25 A27
  constraint tangent A28 L47
  constraint tangent L26 A29
  constraint collinear L47 L48
  constraint tangent L46 A49
  constraint tangent L48 A49
  constraint tangent L45 A50
  constraint tangent L47 A50
  constraint equal A49 A50
  measures "d213" distance of L17 L30
  measures "d214" distance of L20 L44
  measures "d215" radius of A47
  measures "d216" distance of L0 L36
  measures "d217" distance of L9 L48
  measures "d218" radius of A49
extrude "Extrude1'''" add sketch "label outline" along normal blind 0.1 separate body makes body 4 in component "Label"
fillet "Fillet13" radius 2 8 edges at (26.5, 57.5, -6.4) (62.6213, 56.6213, -6.4) (63.5, 28.75, -6.4) (62.6213, 0.8787, -6.4) (26.5, 0, -6.4) (-9.6213, 0.8787, -6.4) (-10.5, 28.75, -6.4) (-9.6213, 56.6213, -6.4) on bodies 2 in component "diag_up_bottom_noVM"
component "PCB" placed x (1, 0, 0) y (0, 1, 0) z (0, 0, 1) at (0, 0, 0)
component "diag_up_bottom_noVM" placed x (1, 0, 0) y (0, 1, 0) z (0, 0, 1) at (0, 0, 0)
component "diag_up_top_noVM" placed x (1, 0, 0) y (0, 1, 0) z (0, 0, 1) at (0, 0, 0)
component "Label" placed x (1, 0, 0) y (0, 1, 0) z (0, 0, 1) at (0, 0, 0)
equation "pcb_thickness = 1.6 mm"
equation "below = 2.8 mm + pcb_thickness"
equation "wall = 2 mm"
equation "width = 70 mm + 2 * wall"
equation "length = pcb_length + 0.5 mm + wall"
equation "above = 10 mm - wall"
equation "pcb_width = 53 mm"
equation "pcb_length = 55 mm"
equation "r_corner = 3 mm"
equation "drill = 3.5 mm"
equation "d_screw = 7 mm"
equation "tol_x = 0.3 mm"
equation "tol_connector = 0.6 mm"
equation "d_post = 8.5 mm"
equation "d_post2 = 8 mm"
equation "bottom_height = 4.3 mm + below"
equation "overlap = 1 mm"
equation "top_height = above + below - bottom_height - tol_y"
equation "d34 = -below"
equation "d35 = tol_connector"
equation "d37 = d35"
equation "d47 = length"
equation "d48 = r_corner"
equation "d49 = ( width - pcb_width ) / 2"
equation "d50 = width"
equation "d51 = wall"
equation "d53 = drill"
equation "d54 = d_screw"
equation "d56 = drill"
equation "d57 = d_screw"
equation "d58 = d_post"
equation "d59 = ( width - pcb_width - 2 * wall ) / 4"
equation "d60 = d59"
equation "d61 = drill"
equation "d64 = tol_x"
equation "d65 = tol_x"
equation "d66 = drill"
equation "d67 = d59"
equation "d68 = d67"
equation "d71 = d_post"
equation "d72 = wall * 0.6"
equation "d73 = -wall"
equation "d77 = bottom_height + overlap"
equation "d79 = bottom_height"
equation "d81 = below - pcb_thickness"
equation "d83 = below"
equation "d88 = tol_x"
equation "d89 = d86"
equation "d90 = d87"
equation "d91 = tol_x"
equation "d98 = above"
equation "d100 = wall * 0.4"
equation "d105 = d_screw"
equation "d106 = d_screw"
equation "d107 = d_screw"
equation "d108 = d_screw"
equation "d109 = tol_connector"
equation "d110 = tol_connector"
equation "d111 = tol_connector"
equation "d112 = tol_connector"
equation "d113 = tol_connector"
equation "d114 = tol_connector"
equation "d115 = tol_connector"
equation "d116 = tol_connector"
equation "d117 = tol_connector"
equation "d118 = tol_connector"
equation "d119 = tol_connector"
equation "d120 = tol_connector"
equation "d126 = -above + tol_y"
equation "d128 = -above + tol_y"
equation "d130 = -top_height + overlap"
equation "d132 = -top_height"
equation "d138 = -top_height - 1.5 mm"
equation "tol_y = 0.2 mm"
equation "d143 = d142"
equation "d144 = d142"
equation "d145 = d142"
equation "d146 = d142"
equation "d147 = d142"
equation "d148 = d142"
equation "d149 = d142"
equation "d150 = wall / 2"
equation "d153 = wall / 4"
equation "d195 = d194"
equation "d196 = d194"
equation "d200 = d199"
equation "d201 = d199"
named bodies: "PCB", "top shell", "label"
